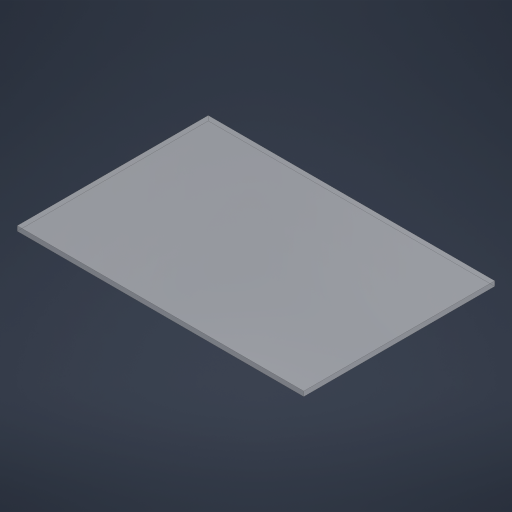
# Autodesk Inventor part: Battery-Holder
Saved by Autodesk Inventor 2024 (Build 280153000, 153)
## iProperties
Created: 2024-01-21
Part Number: Battery-Holder
Material: Polycarbonate, Clear
Document SubType Name: Sheet Metal
Designer: abhin
Density: 1.2 g/cm^3
Flat Pattern Width: 6.35 cm
Flat Pattern Length: 9.525 cm
Flat Pattern Area: 60.4837 cm^2
Sheet Metal Rule: Default
Sheet Metal Width: 2.500 in
Sheet Metal Length: 3.750 in
Sheet Metal Area: 9.375 in^2
Appearance: Polycarbonate - Clear
Author: abhin
Autodesk Inventor part; units mm, degrees
ref_plane "YZ Plane" through (0, 0, 0) normal (1, 0, 0) x (0, 1, 0)
ref_plane "XZ Plane" through (0, 0, 0) normal (0, 1, 0) x (-1, 0, 0)
ref_plane "XY Plane" through (0, 0, 0) normal (0, 0, 1) x (1, 0, 0)
sketch "Sketch1" plane through (0, 0, 0) normal (0, 1, 0) x (-1, 0, 0)
  line L0 (47.625, 31.75) -> (-47.625, 31.75)
  line L1 (-47.625, 31.75) -> (-47.625, -31.75)
  line L2 (-47.625, -31.75) -> (47.625, -31.75)
  line L3 (47.625, -31.75) -> (47.625, 31.75)
  line L4 (47.625, 31.75) -> (-47.625, -31.75) construction
  line L5 (-47.625, 31.75) -> (47.625, -31.75) construction
  point P0 (0, 0)
  dimension "d0" = 95.25
  dimension "d1" = 63.5
  constraints: 12 end point, 2 midpoint, 2 parallel, 1 horizontal, 1 perpendicular
  measures "d0" distance of L2.end L1.end
  measures "d1" distance of L1.end L0.end
extrude "Extrusion1" add sketch "Sketch1" along normal blind 1.5875
equation "\"BendRadius\" = Thickness"
equation "\"BendReliefWidth\" = Thickness"
equation "\"BendReliefDepth\" = 0.5 * Thickness"
equation "\"CornerReliefSize\" = 4 * Thickness"
equation "\"MinimumRemnant\" = 2 * Thickness"
equation "\"TransitionRadius\" = BendRadius"
equation "\"JacobiRadiusSize\" = BendRadius"
equation "\"GapSize\" = Thickness"
equation "\"Thickness\" = 1.5875"
body "Solid1"
